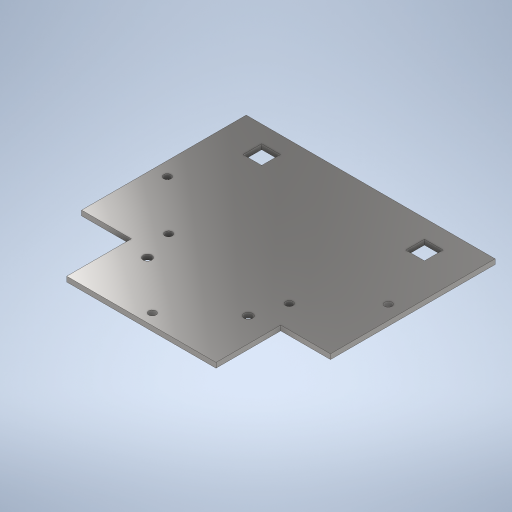
# Autodesk Inventor part: podstawa
Saved by Autodesk Inventor 2023 (Build 270158000, 158)
## iProperties
Created: 2023-07-07
Part Number: podstawa
Material: Stal, węglowa
Document SubType Name: Modeling
Designer: Kamil
Density: 7.85 g/cm^3
Appearance: Częściowo polerowany
Mass: 124.539 g
Surface Area: 169.268 cm^2
Volume: 15.8648 cm^3
Author: Kamil
Autodesk Inventor part; units mm, degrees
ref_plane "YZ Plane" through (0, 0, 0) normal (1, 0, 0) x (0, 1, 0)
ref_plane "XZ Plane" through (0, 0, 0) normal (0, 1, 0) x (-1, 0, 0)
ref_plane "XY Plane" through (0, 0, 0) normal (0, 0, 1) x (1, 0, 0)
sketch "Szkic1" plane through (0, 0, 0) normal (0, 1, 0) x (-1, 0, 0)
  circle A0 centre (45.7688, -11.3479) radius 1.5
  circle A1 centre (25.5188, -29.6192) radius 1.75
  circle A2 centre (66.0188, -29.6192) radius 1.75
  line L0 (-4.2312, -99.4192) -> (95.7688, -99.4192)
  line L1 (95.7688, -99.4192) -> (95.7688, -32.9192)
  line L2 (95.7688, -32.9192) -> (75.7688, -32.9192)
  line L3 (75.7688, -32.9192) -> (75.7688, -6.9192)
  line L4 (75.7688, -6.9192) -> (15.7688, -6.9192)
  line L5 (15.7688, -6.9192) -> (15.7688, -32.9192)
  line L6 (15.7688, -32.9192) -> (-4.2312, -32.9192)
  line L7 (-4.2312, -32.9192) -> (-4.2312, -99.4192)
  point P0 (0, 0)
  point P1 (0, 0)
  constraints: 16 end point, 3 centre point
extrude "Wyciągnięcie proste1" add sketch "Szkic1" along normal blind 2
sketch "Szkic2" plane through (0, 0, 0) normal (0, -1, 0) x (1, 0, 0)
  circle A0 centre (-1.3688, -61.7778) radius 1.5 projected
  circle A1 centre (-21.5202, -42.1278) radius 1.5 projected
  circle A2 centre (-70.0174, -42.1278) radius 1.5 projected
  circle A3 centre (-90.1688, -61.7778) radius 1.5 projected
  point P0 (0, 0)
extrude "Wyciągnięcie proste2" cut sketch "Szkic2" against normal blind 2
sketch "Szkic3" plane through (4.2312, 0, -32.9192) normal (1, 0, 0) x (0, 0, -1)
  line L0 (0, 0) -> (66.5, 0) projected
  line L1 (66.5, 0) -> (66.5, 2) projected
  line L2 (0, 2) -> (66.5, 2) projected
  line L3 (0, 0) -> (0, 2) projected
  line L4 (46.3508, 37) -> (66.9119, -1.4451) projected
  point P0 (-32.9192, 0)
  point P1 (65.0694, 2)
  point P2 (66.1391, 0)
extrude "Wyciągnięcie proste3" cut sketch "Szkic3" against normal through all contours L4 L2 L1 L0
sketch "Szkic4" plane through (0, 0, 0) normal (0, -1, 0) x (1, 0, 0)
  circle A0 centre (-11.7244, -89.168) radius 0.3048 projected
  circle A1 centre (-14.2644, -89.168) radius 0.3048 projected
  circle A2 centre (-14.2644, -86.628) radius 0.3048 projected
  circle A3 centre (-11.7244, -86.628) radius 0.3048 projected
  circle A4 centre (-80.1774, -89.676) radius 0.3048 projected
  circle A5 centre (-77.6374, -89.676) radius 0.3048 projected
  circle A6 centre (-77.6374, -87.136) radius 0.3048 projected
  circle A7 centre (-80.1774, -87.136) radius 0.3048 projected
  line L0 (-11.7244, -86.628) -> (-14.2644, -86.628)
  line L1 (-14.2644, -86.628) -> (-14.2644, -89.168)
  line L2 (-14.2644, -89.168) -> (-11.7244, -89.168)
  line L3 (-11.7244, -89.168) -> (-11.7244, -86.628)
  line L4 (-77.6374, -87.136) -> (-80.1774, -87.136)
  line L5 (-80.1774, -87.136) -> (-80.1774, -89.676)
  line L6 (-80.1774, -89.676) -> (-77.6374, -89.676)
  line L7 (-77.6374, -89.676) -> (-77.6374, -87.136)
  circle A8 centre (-78.9074, -88.406) radius 3.75
  circle A9 centre (-12.9944, -87.898) radius 3.75
  line L8 (-16.7444, -84.148) -> (-9.2444, -84.148)
  line L9 (-9.2444, -84.148) -> (-9.2444, -91.648)
  line L10 (-9.2444, -91.648) -> (-16.7444, -91.648)
  line L11 (-16.7444, -91.648) -> (-16.7444, -84.148)
  line L12 (-82.6574, -84.656) -> (-75.1574, -84.656)
  line L13 (-75.1574, -84.656) -> (-75.1574, -92.156)
  line L14 (-75.1574, -92.156) -> (-82.6574, -92.156)
  line L15 (-82.6574, -92.156) -> (-82.6574, -84.656)
  point P0 (0, 0)
  dimension "d6" = 7.5
  dimension "d7" = 7.5
  constraints: 32 end point, 8 parallel, 4 horizontal, 4 perpendicular, 2 centre point
  measures "d6" diameter of A8
  measures "d7" diameter of A9
extrude "Wyciągnięcie proste4" cut sketch "Szkic4" against normal through all contours A0 L2 L3 | L3 L2 A0 | A0 L2 A1 L1 A2 L0 A3 L3 | L3 L0 A3 | A3 L0 L3 | L2 L1 A1 | A1 L1 L2 | L0 L1 A2 | A2 L1 L0 | L6 L5 A4 | A4 L5 L6 | A4 L5 A7 L4 A6 L7 A5 L6 | L6 L7 A5 | A5 L7 L6 | L5 L4 A7 | A7 L4 L5 | L7 L4 A6 | A6 L4 L7 | A8 | L13 L14 A8 | A8 L12 L13 | A8 L15 L12 | L14 L15 A8 | A9 | L9 L10 A9 | A9 L8 L9 | A9 L11 L8 | L10 L11 A9
sketch "Szkic6" plane through (4.2312, 2, -32.9192) normal (1, 0, 0) x (0, 0, -1)
  line L0 (66.1391, -2) -> (65.0694, 0) projected
  line L1 (0, 0) -> (65.0694, 0) projected
  line L2 (0, -2) -> (0, 0) projected
  line L3 (66.1391, 0) -> (65, 0)
  line L4 (65, 0) -> (65, -3)
  line L5 (65, -3) -> (66.1391, -3)
  line L6 (66.1391, -3) -> (66.1391, 0)
  line L7 (0, -2) -> (66.1391, -2) projected
  point P0 (-32.9192, -2)
  constraints: 8 end point, 2 parallel, 1 horizontal, 1 perpendicular
extrude "Wyciągnięcie proste6" add sketch "Szkic6" against normal blind 100 contours L0 L3 L6
